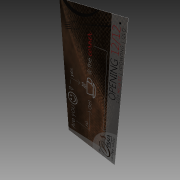
# Autodesk Inventor part: Part1
Saved by Autodesk Inventor 2015 (Build 190159000, 159)
## iProperties
Created: 2015-11-07
Part Number: Part1
Material: Generic
Document SubType Name: Modeling
Designer: Brian
Density: 1 g/cm^3
Appearance: Default
Author: Brian
Autodesk Inventor part; units mm, degrees
ref_plane "YZ Plane" through (0, 0, 0) normal (1, 0, 0) x (0, 1, 0)
ref_plane "XZ Plane" through (0, 0, 0) normal (0, 1, 0) x (-1, 0, 0)
ref_plane "XY Plane" through (0, 0, 0) normal (0, 0, 1) x (1, 0, 0)
sketch "Sketch1" plane through (0, 0, 0) normal (0, 1, 0) x (-1, 0, 0)
  line L0 (0, 0) -> (99, 0)
  line L1 (99, 0) -> (99, -210)
  line L2 (99, -210) -> (0, -210)
  line L3 (0, -210) -> (0, 0)
  dimension "d0" = 99
  dimension "d1" = 210
  constraints: 8 end point, 2 parallel, 1 horizontal, 1 perpendicular
  measures "d0" distance of L1.end L2.end
  measures "d1" distance of L0.end L1.end
extrude "Extrusion1" add sketch "Sketch1" along normal blind 0.5
sketch "Sketch2" plane through (0, 0.5, 0) normal (0, 1, 0) x (1, 0, 0)
  line L0 (-98.9901, -0.0047) -> (-99, 210) construction
  line L1 (-99, 210) -> (-0.0099, 210.0047) construction
  line L2 (-0.0099, 210.0047) -> (0, 0) construction
  line L3 (0, 0) -> (-98.9901, -0.0047) construction
  constraints: 2 coincident, 2 other
sketch "Sketch3" plane through (0, 0, 0) normal (0, -1, 0) x (1, 0, 0)
  line L0 (-99, -210) -> (-98.9901, 0.0047) construction
  line L1 (-98.9901, 0.0047) -> (0, 0) construction
  line L2 (0, 0) -> (-0.0099, -210.0047) construction
  line L3 (-0.0099, -210.0047) -> (-99, -210) construction
  constraints: 2 coincident, 2 other
decal "Decal1"
decal "Decal2"
body "Solid1"
